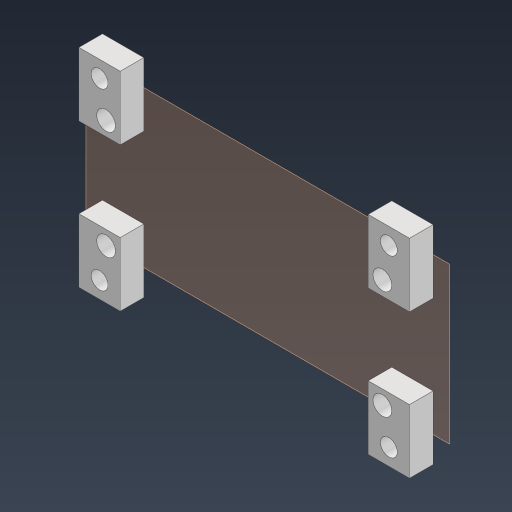
# Autodesk Inventor part: my_pcb_holder
Saved by Autodesk Inventor 2023 (Build 270158000, 158)
## iProperties
Created: 2026-01-23
Part Number: my_pcb_holder
Material: Generic
Document SubType Name: Modeling
Designer: szymo
Density: 1 g/cm^3
Appearance: Default
Author: szymo
Autodesk Inventor part; units mm, degrees
ref_plane "YZ Plane" through (0, 0, 0) normal (1, 0, 0) x (0, 1, 0)
ref_plane "XZ Plane" through (0, 0, 0) normal (0, 1, 0) x (-1, 0, 0)
ref_plane "XY Plane" through (0, 0, 0) normal (0, 0, 1) x (1, 0, 0)
ref_plane "Work Plane1" through (0, 0, 0) normal (0, 0, 1) x (1, 0, 0)
sketch "Sketch1" plane through (0, 0, 0) normal (0, 0, 1) x (1, 0, 0)
  line L0 (-35, 15) -> (-35, -15) projected
  line L1 (-35, -15) -> (35, -15) projected
  line L2 (35, -15) -> (35, 15) projected
  line L3 (35, 15) -> (-35, 15) projected
  circle A0 centre (29.25, 11.5) radius 1.5 projected
  circle A1 centre (29.25, -11.5) radius 1.5 projected
  circle A2 centre (-29.25, 11.5) radius 1.5 projected
  circle A3 centre (-29.25, -11.5) radius 1.5 projected
  line L4 (35, 8.5) -> (26.25, 8.5)
  line L5 (26.25, 8.5) -> (26.25, 22)
  line L6 (26.25, 22) -> (35, 22)
  line L7 (35, 22) -> (35, 8.5)
  line L8 (35, -8.5) -> (26.25, -8.5)
  line L9 (26.25, -8.5) -> (26.25, -22)
  line L10 (26.25, -22) -> (35, -22)
  line L11 (35, -22) -> (35, -8.5)
  line L12 (-35, 8.5) -> (-26.25, 8.5)
  line L13 (-26.25, 8.5) -> (-26.25, 22)
  line L14 (-26.25, 22) -> (-35, 22)
  line L15 (-35, 22) -> (-35, 8.5)
  line L16 (-35, -8.5) -> (-26.25, -8.5)
  line L17 (-26.25, -8.5) -> (-26.25, -22)
  line L18 (-26.25, -22) -> (-35, -22)
  line L19 (-35, -22) -> (-35, -8.5)
  point P0 (0, 0)
  dimension "d0" = 3
  dimension "d1" = 3
  dimension "d2" = 7
  dimension "d3" = 3
  dimension "d4" = 3
  dimension "d5" = 7
  dimension "d6" = 7
  dimension "d7" = 3
  dimension "d8" = 3
  dimension "d9" = 3
  dimension "d10" = 3
  dimension "d11" = 7
  constraints: 32 end point, 8 parallel, 4 horizontal, 4 perpendicular, 4 point on line
  measures "d0" distance from line of L5 A0.centre
  measures "d1" distance from line of A0.centre L4
  measures "d2" distance between parallel lines of L6 L3
  measures "d3" distance from line of L9 A1.centre
  measures "d4" distance from line of L8 A1.centre
  measures "d5" distance between parallel lines of L1 L10
  measures "d6" distance between parallel lines of L14 L3
  measures "d7" distance from line of L13 A2.centre
  measures "d8" distance from line of L12 A2.centre
  measures "d9" distance from line of L16 A3.centre
  measures "d10" distance from line of L17 A3.centre
  measures "d11" distance between parallel lines of L1 L18
extrude "Extrusion1" add sketch "Sketch1" along normal blind 5 contours L3 L13 L12 L0 | L15 L14 L13 L3 | L16 L17 L1 L0 | L5 L6 L7 L3 | L3 L2 L4 L5 | L1 L17 L18 L19 | L9 L8 L2 L1 | L1 L11 L10 L9 | A0 | A1 | A2 | A3
sketch "Sketch2" plane through (0, 0, 0) normal (0, 0, -1) x (-1, 0, 0)
  line L0 (-22.6874, -6.3823) -> (-22.6874, 8.2103) projected
  line L1 (-22.6874, 8.2103) -> (19.4692, 8.2103) projected
  line L2 (19.4692, 8.2103) -> (19.4692, -6.3823) projected
  line L3 (19.4692, -6.3823) -> (-22.6874, -6.3823) projected
  line L4 (35, 15) -> (35, -15) projected
  line L5 (-35, 15) -> (35, 15) projected
  line L6 (-35, -15) -> (-35, 15) projected
  line L7 (35, -15) -> (-35, -15) projected
  circle A0 centre (-29.25, 11.5) radius 1.5 projected
  circle A1 centre (-29.25, -11.5) radius 1.5 projected
  circle A2 centre (29.25, 11.5) radius 1.5 projected
  circle A3 centre (29.25, -11.5) radius 1.5 projected
  point P0 (0, 0)
  constraints: 4 coincident
hole "Hole1" at (29.25, 11.5, 0) at (29.25, -11.5, 0) at (-29.25, -11.5, 0) at (-29.25, 11.5, 0) direction (0, 0, 1) diameter 4 depth 5 counterbore diameter 4.5 counterbore depth 0.5
sketch "Sketch3" plane through (0, 0, 0) normal (0, 0, -1) x (-1, 0, 0)
  circle A0 centre (29.25, 11.5) radius 2.25 projected
  line L0 (26.25, 22) -> (35, 22) projected
  line L1 (26.25, 8.5) -> (26.25, 22) projected
  line L2 (35, 8.5) -> (26.25, 8.5) projected
  line L3 (35, 22) -> (35, 8.5) projected
  circle A1 centre (29.25, -11.5) radius 2.25 projected
  line L4 (26.25, -8.5) -> (35, -8.5) projected
  line L5 (26.25, -22) -> (26.25, -8.5) projected
  line L6 (35, -22) -> (26.25, -22) projected
  line L7 (35, -8.5) -> (35, -22) projected
  circle A2 centre (-29.25, -11.5) radius 2.25 projected
  line L8 (-26.25, -22) -> (-35, -22) projected
  line L9 (-26.25, -8.5) -> (-26.25, -22) projected
  line L10 (-35, -8.5) -> (-26.25, -8.5) projected
  line L11 (-35, -22) -> (-35, -8.5) projected
  circle A3 centre (-29.25, 11.5) radius 2.25 projected
  line L12 (-26.25, 8.5) -> (-35, 8.5) projected
  line L13 (-26.25, 22) -> (-26.25, 8.5) projected
  line L14 (-35, 22) -> (-26.25, 22) projected
  line L15 (-35, 8.5) -> (-35, 22) projected
  line L16 (-22.6874, -6.3823) -> (-22.6874, 8.2103) projected
  line L17 (-22.6874, 8.2103) -> (19.4692, 8.2103) projected
  line L18 (19.4692, 8.2103) -> (19.4692, -6.3823) projected
  line L19 (19.4692, -6.3823) -> (-22.6874, -6.3823) projected
  line L20 (35, 15) -> (35, -15) projected
  line L21 (-35, 15) -> (35, 15) projected
  line L22 (-35, -15) -> (-35, 15) projected
  line L23 (35, -15) -> (-35, -15) projected
  circle A4 centre (-29.25, 11.5) radius 1.5 projected
  circle A5 centre (-29.25, -11.5) radius 1.5 projected
  circle A6 centre (29.25, 11.5) radius 1.5 projected
  circle A7 centre (29.25, -11.5) radius 1.5 projected
  line L24 (26.25, 22) -> (35, 22) projected
  line L25 (35, 22) -> (26.25, 15.25)
  line L26 (26.25, 8.5) -> (26.25, 22) projected
  line L27 (35, 15) -> (26.25, 22)
  line L28 (26.25, -22) -> (26.25, -8.5) projected
  line L29 (26.25, -22) -> (35, -15)
  line L30 (26.25, -15) -> (35, -22)
  line L31 (-35, 15) -> (-26.25, 22)
  line L32 (-26.25, 22) -> (-26.25, 8.5) projected
  line L33 (-35, 22) -> (-26.25, 22) projected
  line L34 (-26.25, 15) -> (-35, 22)
  line L35 (-26.25, -8.5) -> (-26.25, -22) projected
  line L36 (-26.25, -15.25) -> (-35, -22)
  line L37 (-26.25, -22) -> (-35, -15)
  point P0 (0, 0)
  point P1 (30.625, 18.5)
  point P2 (30.625, -18.5)
  point P3 (-30.625, -18.5)
  point P4 (-30.625, 18.5)
  constraints: 16 end point, 6 midpoint, 4 point on line, 1 parallel
hole "Hole2" at (-30.625, 18.5, 0) at (-30.625, -18.5, 0) at (30.625, -18.5, 0) at (30.625, 18.5, 0) direction (0, 0, 1) diameter 3.6 depth 5 countersink diameter 7 countersink angle 90 clearance for "Countersunk Flat Head Screw ISO 2009/7046" size "M3" standard "ISO"
body "Solid1"
